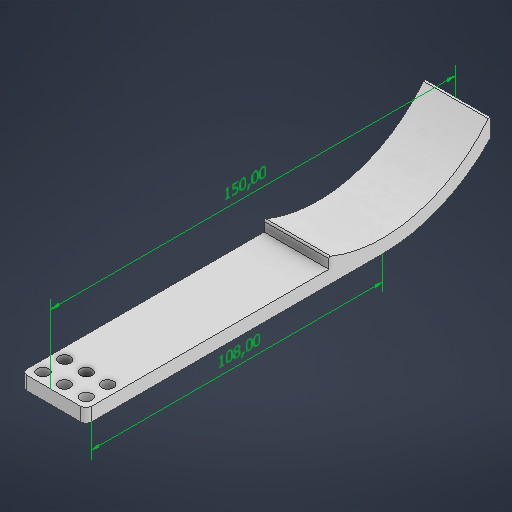
# Autodesk Inventor part: Launcher_Arm_V2
Saved by Autodesk Inventor 2026.1 (Build 301233020, 233B)
## iProperties
Created: 2025-11-02
Part Number: Launcher_Arm_V2
Material: Generic
Document SubType Name: Modeling
Designer: Asus
Density: 1 g/cm^3
Appearance: Default
Author: Asus
Autodesk Inventor part; units mm, degrees
ref_plane "YZ Plane" through (0, 0, 0) normal (1, 0, 0) x (0, 1, 0)
ref_plane "XZ Plane" through (0, 0, 0) normal (0, 1, 0) x (-1, 0, 0)
ref_plane "XY Plane" through (0, 0, 0) normal (0, 0, 1) x (1, 0, 0)
sketch "Sketch1" plane through (0, 0, 0) normal (0, 1, 0) x (-1, 0, 0)
  line L0 (-10, 75) -> (10, 75)
  line L1 (12, 73) -> (12, -75)
  line L2 (12, -75) -> (-12, -75)
  line L3 (-12, -75) -> (-12, 73)
  line L4 (-12, 75) -> (12, -75) construction
  line L5 (12, 75) -> (-12, -75) construction
  arc A0 (12, 73) -> (10, 75) centre (10, 73) ccw
  arc A1 (-10, 75) -> (-12, 73) centre (-10, 73) ccw
  circle A2 centre (8, 71) radius 2.2
  circle A3 centre (0, 71) radius 2.2
  circle A4 centre (-8, 71) radius 2.2
  circle A5 centre (8, 63) radius 2.2
  circle A6 centre (0, 63) radius 2.2
  circle A7 centre (-8, 63) radius 2.2
  point P0 (0, 0)
  dimension "d0" = 24
  dimension "d1" = 150
  dimension "d2" = 2
  dimension "d3" = 4.4
  dimension "d4" = 4
  dimension "d5" = 4
  dimension "d8" = 8
  dimension "d11" = 8
  constraints: 12 end point, 8 centre point, 4 point on circle, 4 point on line, 4 tangent, 2 horizontal, 2 midpoint, 2 parallel, 1 equal radius, 1 perpendicular, 1 vertical, 10 other
  measures "d0" distance of L1.end L2.end
  measures "d1" distance of L5.start L1.end
  measures "d2" radius of A0
  measures "d3" diameter of A2
  measures "d4" distance from line of L1 A2.centre
  measures "d5" distance from line of L0 A2.centre
  measures "d8" distance of A2.centre A3.centre
  measures "d11" distance of A2.centre A5.centre
extrude "Extrusion1" add sketch "Sketch1" along normal blind 5
sketch "Sketch2" plane through (12, 0, 73) normal (1, 0, 0) x (0, 0, -1)
  arc A0 (108, 5) -> (147.1089, 23.8473) centre (108, 55) ccw
  line L0 (0, 5) -> (148, 5) projected
  line L1 (148, 5) -> (148, 23.5357)
  arc A1 (148, 23.5357) -> (147.1089, 23.8473) centre (147.5, 23.5357) ccw
  point P0 (73, 0)
  point P1 (148, 25)
  dimension "d16" = 100
  dimension "d17" = 40
  dimension "d18" = 0.5
  constraints: 5 point on circle, 3 tangent, 2 centre point, 2 end point, 2 point on line, 1 vertical
  measures "d16" diameter of A0
  measures "d17" distance from line of L1 A0.centre
  measures "d18" radius of A1
extrude "Extrusion2" add sketch "Sketch2" against normal blind 24
sketch "Sketch3" plane through (12, 0, 73) normal (1, 0, 0) x (0, 0, -1)
  line L0 (0, 0) -> (148, 0) projected
  arc A0 (108, 5) -> (147.1089, 23.8473) centre (108, 55) ccw projected
  line L1 (0, 5) -> (108, 5) projected
  arc A1 (108, 0) -> (147.8624, 17.1055) centre (108, 55) ccw
  line L2 (148, 0) -> (148, 23.5357) projected
  line L3 (148, 17.2508) -> (148, 0)
  line L4 (148, 0) -> (108, 0)
  arc A2 (147.8624, 17.1055) -> (148, 17.45) centre (147.5, 17.45) ccw
  point P0 (150, 0)
  dimension "d27" = 1
  dimension "d28" = 17.2508
  constraints: 4 end point, 4 point on circle, 3 tangent, 2 centre point, 2 point on line, 1 coincident, 1 vertical
  measures "d27" diameter of A2
  measures "d28" distance of L0.end L3.start
extrude "Extrusion3" cut sketch "Sketch3" against normal blind 24
sketch "Sketch4" plane through (12, 0, 73) normal (1, 0, 0) x (0, 0, -1)
  arc A0 (88.6931, 8.878) -> (108, 5) centre (108, 55) ccw
  line L0 (0, 5) -> (108, 5) projected
  line L1 (148, 17.45) -> (148, 23.5357) projected
  line L2 (88, 5) -> (88, 8.4167)
  arc A1 (88.6931, 8.878) -> (88, 8.4167) centre (88.5, 8.4167) ccw
  point P0 (73, 0)
  point P1 (88, 9.1742)
  dimension "d31" = 0.5
  dimension "d40" = 20
  dimension "d41" = 50
  constraints: 5 point on circle, 3 end point, 3 tangent, 2 centre point, 2 point on line, 1 perpendicular
  measures "d31" radius of A1
  measures "d40" distance from line of L0.end L2
  measures "d41" radius of A0
extrude "Extrusion4" add sketch "Sketch4" against normal blind 24
body "Solid1"
